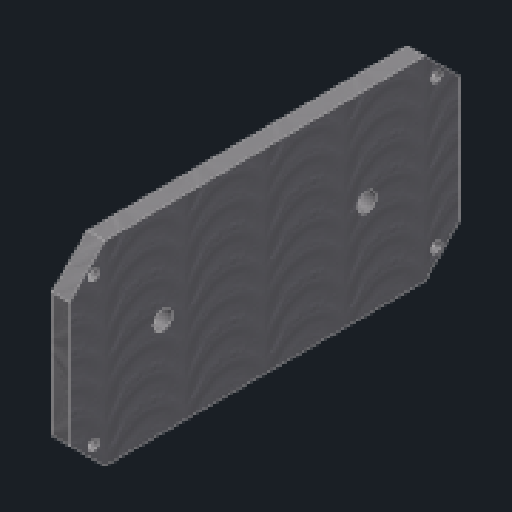
# Autodesk Inventor part: CAJA
Saved by Autodesk Inventor 2024.3 (Build 283343000, 343)
## iProperties
Created: 2024-06-29
Part Number: CAJA
Material: Steel, Mild, Welded
Document SubType Name: Modeling
Designer: Niler
Density: 7.85 g/cm^3
Appearance: Weld - Steel Mild
Author: Niler
Autodesk Inventor part; units mm, degrees
ref_plane "YZ Plane" through (0, 0, 0) normal (1, 0, 0) x (0, 1, 0)
ref_plane "XZ Plane" through (0, 0, 0) normal (0, 1, 0) x (-1, 0, 0)
ref_plane "XY Plane" through (0, 0, 0) normal (0, 0, 1) x (1, 0, 0)
sketch "Sketch1" plane through (0, 0, 0) normal (1, 0, 0) x (0, 1, 0)
  line L0 (-55, 110) -> (55, 110)
  line L1 (55, 110) -> (55, -110)
  line L2 (55, -110) -> (-55, -110)
  line L3 (-55, -110) -> (-55, 110)
  line L4 (-55, 110) -> (55, -110) construction
  line L5 (55, 110) -> (-55, -110) construction
  circle A0 centre (0, 57.5) radius 5.3
  circle A1 centre (0, -57.5) radius 5.3
  circle A2 centre (0, 0) radius 5.3
  line L6 (0, 57.5) -> (0, -57.5) construction
  line L7 (45, -100) -> (45, 100)
  line L8 (45, 100) -> (-45, 100)
  line L9 (-45, 100) -> (-45, -100)
  line L10 (-45, -100) -> (45, -100)
  dimension "d0" = 115
  dimension "d1" = 10.6
  dimension "d2" = 220
  dimension "d3" = 110
  dimension "d4" = 10
  constraints: 22 end point, 4 parallel, 3 centre point, 3 midpoint, 2 equal radius, 2 perpendicular, 2 vertical alignment, 1 coincident, 1 horizontal, 1 vertical, 3 other
  measures "d0" distance of L6.end L6.start
  measures "d1" diameter of A0
  measures "d2" distance between parallel lines of L2 L0
  measures "d3" distance of L0.start L0.end
  measures "d4" distance between parallel lines of L1 L7
extrude "Extrusion1" add sketch "Sketch1" along normal blind 10 contours L0 L1 L2 L3 | A2 | L10 L9 L8 L7
chamfer "Chamfer2" distance 20 angle 45 4 edges at (5, 55, -110) (5, -55, -110) (5, -55, 110) (5, 55, 110)
sketch "Sketch3" plane through (0, 0, 0) normal (-1, 0, 0) x (0, 0, 1)
  circle A0 centre (0, 0) radius 7.5
  dimension "d16" = 15
  constraints: 1 centre point, 1 coincident
  measures "d16" diameter of A0
extrude "Extrusion3" cut sketch "Sketch3" against normal blind 7
sketch "Sketch5" plane through (10, 0, 0) normal (1, 0, 0) x (0, 0, -1)
  circle A0 centre (96.5, -41.5) radius 1.5 projected
  circle A1 centre (-96.5, -41.5) radius 1.5 projected
  circle A2 centre (96.5, 41.5) radius 1.5 projected
  circle A3 centre (-96.5, 41.5) radius 1.5 projected
  line L0 (110, 35) -> (90, 55) projected
  line L1 (110, 35) -> (110, -35) projected
  line L2 (90, -55) -> (110, -35) projected
  line L3 (90, -55) -> (-90, -55) projected
  line L4 (-110, -35) -> (-90, -55) projected
  line L5 (-110, -35) -> (-110, 35) projected
  line L6 (-90, 55) -> (-110, 35) projected
  line L7 (-90, 55) -> (90, 55) projected
  circle A4 centre (0, 0) radius 10.3 projected
  circle A5 centre (33.234, -33.234) radius 2.75 projected
  circle A6 centre (33.234, 33.234) radius 2.75 projected
  circle A7 centre (-33.234, -33.234) radius 2.75 projected
  circle A8 centre (-33.234, 33.234) radius 2.75 projected
  point P0 (0, 0)
extrude "Extrusion4" cut sketch "Sketch5" against normal through all contours A0 | A1 | A2 | A3
sketch "Sketch6" plane through (10, 0, 0) normal (1, 0, 0) x (0, 0, -1)
  circle A0 centre (96.5, -41.5) radius 1.5 projected
  circle A1 centre (-96.5, -41.5) radius 1.5 projected
  circle A2 centre (96.5, 41.5) radius 1.5 projected
  circle A3 centre (-96.5, 41.5) radius 1.5 projected
  line L0 (-110, 35) -> (-90, 55) projected
  line L1 (-110, 35) -> (-110, -35) projected
  line L2 (-90, -55) -> (-110, -35) projected
  line L3 (-90, -55) -> (90, -55) projected
  line L4 (110, -35) -> (90, -55) projected
  line L5 (110, -35) -> (110, 35) projected
  line L6 (90, 55) -> (110, 35) projected
  line L7 (90, 55) -> (-90, 55) projected
  circle A4 centre (-57.5, 0) radius 5.3 projected
  circle A5 centre (57.5, 0) radius 5.3 projected
  circle A6 centre (-96.5, 41.5) radius 2.9
  circle A7 centre (-96.5, -41.5) radius 2.9
  circle A8 centre (96.5, -41.5) radius 2.9
  circle A9 centre (96.5, 41.5) radius 2.9
  point P0 (0, 0)
  dimension "d21" = 5.8
  constraints: 4 centre point, 4 coincident, 3 equal radius
  measures "d21" diameter of A6
extrude "Extrusion5" cut sketch "Sketch6" against normal blind 3.5 contours A0 | A1 | A2 | A3 | A6 | A7 | A8 | A9
body "Solid1"
